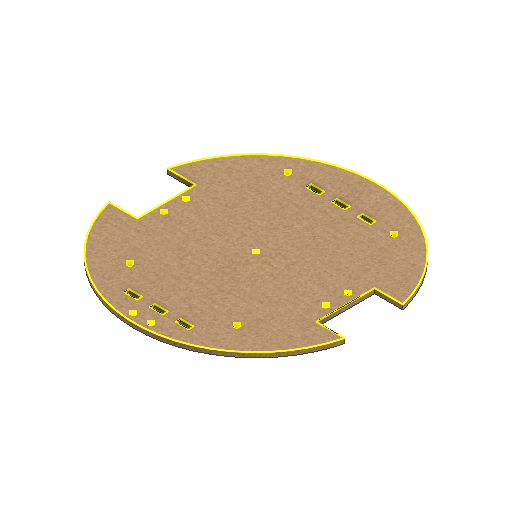
# Autodesk Inventor part: base
Saved by Autodesk Inventor 2025 (Build 290162000, 162)
## iProperties
Created: 2024-09-26
Part Number: base
Material: MDF Medium Density Fiberboard
Document SubType Name: Modeling
Designer: DANIEL
Density: 0.8 g/cm^3
Appearance: Cardboard - Corrugated
Checked By: FERNANDO
Engr Approved By: ANTONIO
Stock Number: 1
Author: DANIEL
Title: BASE
Autodesk Inventor part; units mm, degrees
ref_plane "YZ Plane" through (0, 0, 0) normal (1, 0, 0) x (0, 1, 0)
ref_plane "XZ Plane" through (0, 0, 0) normal (0, 1, 0) x (-1, 0, 0)
ref_plane "XY Plane" through (0, 0, 0) normal (0, 0, 1) x (1, 0, 0)
sketch "Sketch1" plane through (0, 0, 0) normal (0, 1, 0) x (-1, 0, 0)
  circle A0 centre (0, 0) radius 100
  line L0 (0, -140) -> (0, 140) projected
  line L1 (-146.2506, 0) -> (146.2506, 0) projected
  circle A1 centre (7.25, 93.75) radius 1.5
  circle A2 centre (-7.25, 93.75) radius 1.5
  circle A3 centre (-44, 60) radius 1.7
  circle A4 centre (-44, -70) radius 1.7
  circle A5 centre (44, 60) radius 1.7
  circle A6 centre (44, -70) radius 1.7
  circle A7 centre (-67, 9) radius 1.25
  circle A8 centre (-67, -9) radius 1.25
  circle A9 centre (67, 9) radius 1.25
  circle A10 centre (67, -9) radius 1.25
  line L2 (-95.8, 24) -> (-73.8, 24)
  line L3 (-73.8, 24) -> (-73.8, -24)
  line L4 (-73.8, -24) -> (-95.8, -24)
  line L5 (-95.8, -24) -> (-95.8, 24)
  line L6 (-95.8, 24) -> (-104.4647, 24)
  line L7 (-104.4647, 24) -> (-104.4647, -24)
  line L8 (-104.4647, -24) -> (-95.8, -24)
  line L9 (-95.8, -24) -> (-95.8, 24)
  line L10 (95.8, 24) -> (73.8, 24)
  line L11 (73.8, 24) -> (73.8, -24)
  line L12 (73.8, -24) -> (95.8, -24)
  line L13 (95.8, -24) -> (95.8, 24)
  line L14 (95.8, 24) -> (104.4647, 24)
  line L15 (104.4647, 24) -> (104.4647, -24)
  line L16 (104.4647, -24) -> (95.8, -24)
  line L17 (95.8, -24) -> (95.8, 24)
  line L18 (-26.5, 78) -> (26.5, 78)
  line L19 (26.5, 78) -> (26.5, 82)
  line L20 (26.5, 82) -> (-26.5, 82)
  line L21 (-26.5, 82) -> (-26.5, 78)
  line L22 (-26.5, 78) -> (-15.9, 78)
  line L23 (-15.9, 78) -> (-15.9, 82)
  line L24 (-15.9, 82) -> (-26.5, 82)
  line L25 (-26.5, 82) -> (-26.5, 78)
  line L26 (-5.3, 78) -> (-5.3, 82)
  line L27 (5.3, 78) -> (5.3, 82)
  line L28 (15.9, 78) -> (15.9, 82)
  line L29 (-26.5, -72) -> (26.5, -72)
  line L30 (26.5, -68) -> (-26.5, -68)
  line L31 (15.9, -72) -> (15.9, -68)
  line L32 (26.5, -72) -> (26.5, -68)
  line L33 (5.3, -72) -> (5.3, -68)
  line L34 (-5.3, -72) -> (-5.3, -68)
  line L35 (-15.9, -72) -> (-15.9, -68)
  line L36 (-26.5, -68) -> (-26.5, -72)
  point P0 (97.0773, 24)
  point P1 (-97.0773, 24)
  point P2 (-97.0773, -24)
  point P3 (97.0773, -24)
  dimension "diam" = 200
  dimension "d3" = 7.25
  dimension "d4" = 7.25
  dimension "d5" = 93.75
  dimension "d6" = 93.75
  dimension "d7" = 3
  dimension "d8" = 3
  dimension "d9" = 60
  dimension "d10" = 3.4
  dimension "d13" = 130
  dimension "d16" = 88
  dimension "d19" = 44
  dimension "d20" = 67
  dimension "d21" = 9
  dimension "d22" = 2.5
  dimension "d25" = 18
  dimension "d28" = 134
  dimension "d31" = 95.8
  dimension "d32" = 24
  dimension "d33" = 22
  dimension "d34" = 48
  dimension "d35" = 78
  dimension "d36" = 26.5
  dimension "d37" = 53
  dimension "d38" = 4
  dimension "d39" = 10.6
  dimension "d40" = 4
  dimension "d43" = 10.6
  dimension "d50" = 150
  dimension "d55" = 0
  constraints: 70 end point, 11 centre point, 11 coincident, 8 parallel, 8 symmetric about line, 7 horizontal, 4 perpendicular, 3 vertical, 47 other
  measures "diam" diameter of A0
  measures "d3" distance from line of L0 point (-7.25, 93.75)
  measures "d4" distance from line of L0 point (7.25, 93.75)
  measures "d5" distance from line of L1 point (-7.25, 93.75)
  measures "d6" distance from line of L1 point (7.25, 93.75)
  measures "d7" diameter of A1
  measures "d8" diameter of A2
  measures "d9" distance from line of L1 point (-44, 60)
  measures "d10" diameter of A3
  measures "d13" distance of A3.centre A4.centre
  measures "d16" distance of A3.centre A5.centre
  measures "d19" distance from line of L0 A3.centre
  measures "d20" distance from line of L0 point (-67, 9)
  measures "d21" distance from line of L1 point (-67, 9)
  measures "d22" diameter of A7
  measures "d25" distance of A7.centre A8.centre
  measures "d28" distance of A7.centre A9.centre
  measures "d31" distance from line of L0 L2.start
  measures "d32" distance from line of L1 L2.start
  measures "d33" distance of L3.end L4.end
  measures "d34" distance of L2.end L3.end
  measures "d35" distance from line of L1 point (26.5, 78)
  measures "d36" distance from line of L0 point (26.5, 78)
  measures "d37" distance of L20.end L19.end
  measures "d38" distance of L19.end L18.end
  measures "d39" distance of L24.end L23.end
  measures "d40" distance of L23.end L22.end
  measures "d43" distance of L22.end L26.start
  measures "d50" distance of L18.start L29.start
  measures "d55" distance between parallel lines of L4 L8
extrude "Extrusion1" add sketch "Sketch1" along normal blind 4 contours L14 L10 L11 L1 L0 L18 L19 L20 A0 | A0 L0 L29 L32 L30 L1 L11 L12 L16 | L0 L20 L21 L18 L1 L3 L2 L6 A0 | A0 L8 L4 L3 L1 L0 L30 L36 L29 | L20 L28 L18 L27 | L26 L18 L23 L20 | L29 L35 L30 L34 | L33 L30 L31 L29
sketch "Sketch2" plane through (0, 4, 0) normal (0, 1, 0) x (1, 0, 0)
  line L0 (-97.0773, 24) -> (-73.8, 24) projected
  line L1 (-73.8, 24) -> (-73.8, -24) projected
  line L2 (-73.8, -24) -> (-97.0773, -24) projected
  arc A0 (-97.0773, -24) -> (97.0773, -24) centre (0, 0) ccw projected
  line L3 (97.0773, -24) -> (73.8, -24) projected
  line L4 (73.8, -24) -> (73.8, 24) projected
  line L5 (73.8, 24) -> (97.0773, 24) projected
  arc A1 (97.0773, 24) -> (-97.0773, 24) centre (0, 0) ccw projected
  line L6 (15.9, -78) -> (26.5, -78) projected
  line L7 (26.5, -78) -> (26.5, -82) projected
  line L8 (26.5, -82) -> (15.9, -82) projected
  line L9 (15.9, -82) -> (15.9, -78) projected
  line L10 (5.3, 68) -> (-5.3, 68) projected
  line L11 (-5.3, 68) -> (-5.3, 72) projected
  line L12 (-5.3, 72) -> (5.3, 72) projected
  line L13 (5.3, 72) -> (5.3, 68) projected
  line L14 (15.9, 68) -> (15.9, 72) projected
  line L15 (15.9, 72) -> (26.5, 72) projected
  line L16 (26.5, 72) -> (26.5, 68) projected
  line L17 (26.5, 68) -> (15.9, 68) projected
  circle A2 centre (67, 9) radius 1.25 projected
  circle A3 centre (44, 70) radius 1.7 projected
  circle A4 centre (-44, 70) radius 1.7 projected
  circle A5 centre (-67, 9) radius 1.25 projected
  line L18 (-15.9, 72) -> (-15.9, 68) projected
  line L19 (-15.9, 68) -> (-26.5, 68) projected
  line L20 (-26.5, 68) -> (-26.5, 72) projected
  line L21 (-26.5, 72) -> (-15.9, 72) projected
  line L22 (5.3, -78) -> (5.3, -82) projected
  line L23 (5.3, -82) -> (-5.3, -82) projected
  line L24 (-5.3, -82) -> (-5.3, -78) projected
  line L25 (-5.3, -78) -> (5.3, -78) projected
  circle A6 centre (67, -9) radius 1.25 projected
  circle A7 centre (44, -60) radius 1.7 projected
  circle A8 centre (7.25, -93.75) radius 1.5 projected
  line L26 (-15.9, -78) -> (-15.9, -82) projected
  line L27 (-15.9, -82) -> (-26.5, -82) projected
  line L28 (-26.5, -82) -> (-26.5, -78) projected
  line L29 (-26.5, -78) -> (-15.9, -78) projected
  circle A9 centre (-67, -9) radius 1.25 projected
  circle A10 centre (-44, -60) radius 1.7 projected
  circle A11 centre (-7.25, -93.75) radius 1.5 projected
equation "\"d3\" = 0.5 * caster_dist_holes"
equation "\"d4\" = d3"
equation "\"d6\" = d5"
equation "\"d19\" = 0.5 * d16"
equation "\"d25\" = 2 * d21"
equation "\"d28\" = 2 * d20"
equation "\"d34\" = 2 * d32"
equation "\"d39\" = 0.2 * d37"
equation "\"d43\" = d39"
equation "\"caster_dist_holes\" = 14.5"
body "Solid1"
